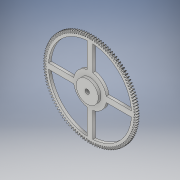
# Autodesk Inventor part: servo-gear
Saved by Autodesk Inventor 2017 (Build 210142000, 142)
## iProperties
Created: 2016-11-23
Part Number: servo-gear
Material: Generic
Document SubType Name: Modeling
Designer: cody
Density: 1 g/cm^3
Appearance: Default
Author: cody
Autodesk Inventor part; units mm, degrees
ref_plane "YZ Plane" through (0, 0, 0) normal (1, 0, 0) x (0, 1, 0)
ref_plane "XZ Plane" through (0, 0, 0) normal (0, 1, 0) x (-1, 0, 0)
ref_plane "XY Plane" through (0, 0, 0) normal (0, 0, 1) x (1, 0, 0)
sketch "Sketch1" plane through (0, 0, 0) normal (0, 0, 1) x (1, 0, 0)
  circle A0 centre (0, 0) radius 25.4
  dimension "d31" = 50.8
  constraints: 1 centre point
  measures "d31" diameter of A0
extrude "Extrusion1" add sketch "Sketch1" along normal blind 1.5875
sketch "Sketch2" plane through (0, 0, 1.5875) normal (0, 0, 1) x (1, 0, 0)
  arc A0 (-50.8, 0) -> (50.8, 0) centre (0, 0) ccw projected
  circle A1 centre (0, 0) radius 1.27
  circle A2 centre (0, 0) radius 6.35
  dimension "d4" = 2.54
  dimension "d5" = 12.7
  constraints: 2 centre point, 2 coincident
  measures "d4" diameter of A1
  measures "d5" diameter of A2
extrude "Extrusion2" add sketch "Sketch2" along normal mid plane 3.175
sketch "Sketch3" plane through (0, 0, 1.5875) normal (0, 0, 1) x (1, 0, 0)
  arc A0 (6.35, 0) -> (6.35, 0) centre (0, 0) ccw projected
  circle A1 centre (0, 0) radius 1.27 projected
  circle A2 centre (0, 0) radius 6.35 construction
  circle A3 centre (0, 0) radius 25.4 projected
  circle A4 centre (0, 0) radius 9.525
  circle A5 centre (0, 0) radius 1.27 projected
  circle A6 centre (0, 0) radius 23.9712
  line L0 (-55.569, 0) -> (51.7908, 0) construction
  line L1 (0, 41.5641) -> (0, -44.9408) construction
  line L2 (-23.9186, 1.5875) -> (-9.3918, 1.5875)
  line L3 (-23.9186, -1.5875) -> (-9.3918, -1.5875)
  line L4 (1.5875, 23.9186) -> (1.5875, 9.3918)
  line L5 (-1.5875, 23.9186) -> (-1.5875, 9.3918)
  line L6 (9.3918, -1.5875) -> (23.9186, -1.5875)
  line L7 (9.3918, 1.5875) -> (23.9186, 1.5875)
  line L8 (1.5875, -9.3918) -> (1.5875, -23.9186)
  line L9 (-1.5875, -9.3918) -> (-1.5875, -23.9186)
  dimension "d32" = 19.05
  dimension "d33" = 47.9425
  dimension "d38" = 50.8
  dimension "d40" = 3.175
  dimension "d41" = 14.5288
  dimension "d42" = 3.175
  dimension "d43" = 14.5268
  dimension "d44" = 3.175
  dimension "d45" = 3.175
  dimension "d46" = 14.5268
  dimension "d47" = 14.5268
  constraints: 20 end point, 8 parallel, 3 coincident, 2 horizontal, 1 centre point, 1 vertical, 21 other
  measures "d38" diameter of A3
  measures "d40" distance between parallel lines of L2 L3
  measures "d42" distance between parallel lines of L4 L5
  measures "d43" distance of L4.start L4.end
  measures "d44" distance of L6.end L7.end
  measures "d45" distance between parallel lines of L9 L8
  measures "d46" distance of L6.start L6.end
  measures "d47" distance of L8.start L8.end
extrude "Extrusion3" cut sketch "Sketch3" against normal blind 1.5875 contours A4 L4 A6 L7 | L6 A6 L8 A4 | A4 L2 A6 L5 | L9 A6 L3 A4
sketch "Sketch4" plane through (0, 0, 1.5875) normal (0, 0, 1) x (1, 0, 0)
  line L0 (0, -30.215) -> (0, -20.5175) construction
  circle A0 centre (0, 0) radius 25.4 projected
  circle A1 centre (0, 0) radius 6.35 projected
  arc A2 (-0.381, -25.3971) -> (0.381, -25.3971) centre (0, 0) ccw
  line L1 (0.127, -30.215) -> (0.127, -20.5175) construction
  line L2 (-0.127, -30.215) -> (-0.127, -20.5175) construction
  circle A3 centre (0, 0) radius 25.4 projected
  line L3 (-0.5678, -26.924) -> (0.7146, -26.924) construction
  line L4 (0.381, -30.215) -> (0.381, -20.5175) construction
  line L5 (-0.381, -30.215) -> (-0.381, -20.5175) construction
  arc A4 (0.1562, -26.8357) -> (0.381, -25.3971) centre (-4.3352, -25.3971) ccw
  line L6 (0, -26.924) -> (0.0353, -26.924)
  arc A5 (0.0353, -26.924) -> (0.1562, -26.8357) centre (0.0353, -26.797) ccw
  arc A6 (-0.381, -25.3971) -> (-0.1562, -26.8357) centre (4.3352, -25.3971) ccw
  line L7 (0, -26.924) -> (-0.0353, -26.924)
  arc A7 (-0.1562, -26.8357) -> (-0.0353, -26.924) centre (-0.0353, -26.797) ccw
  arc A8 (1.5875, -23.9186) -> (23.9186, -1.5875) centre (0, 0) ccw projected
  arc A9 (-0.381, -25.3971) -> (0.381, -25.3971) centre (0, 0) ccw
  point P0 (0.127, -26.924)
  point P1 (-0.127, -26.924)
  dimension "d62" = 0.127
  dimension "d64" = 1.524
  dimension "d65" = 0.254
  dimension "d66" = 0.127
  constraints: 16 end point, 14 point on circle, 10 symmetric about line, 7 point on line, 6 centre point, 3 tangent, 2 coincident, 2 parallel, 2 vertical, 1 collinear, 1 concentric, 1 horizontal, 4 other
  measures "d62" distance between parallel lines of L0 L1
  measures "d64" distance edge to line of A0 L3
  measures "d65" distance between parallel lines of L1 L4
  measures "d66" radius of A5
extrude "Extrusion4" add sketch "Sketch4" against normal blind 1.5875 contours A0 A4 A5 L6 L7 A7 A6
pattern_circular "Circular Pattern2" count 121 over 360 about axis through (0, 0, -10) along (0, 0, 1) of "Extrusion4"
sketch "Sketch6" plane through (0, 0, 3.175) normal (0, 0, 1) x (1, 0, 0)
  circle A0 centre (0, 0) radius 1.27 projected
  circle A1 centre (0, 0) radius 6.35 projected
  dimension "d55" = 2.54
  dimension "d56" = 12.7
  measures "d55" diameter of A0
  measures "d56" diameter of A1
extrude "Extrusion5" cut sketch "Sketch6" against normal through all contours A0
body "Solid1"
